Autodesk Fusion 360 part; units mm, degrees
note: some values were not read from the file. Chosen so that the rebuilt part matches the saved one: which bodies a step acts on.
(part 3 of 4)
ref_plane "WorkPlane163" through (39, 1188.0192, -25.0252) normal (1, 0, 0) x (0, 0, 1)
sketch "Sketch165" plane through (39, 1188.0192, -25.0252) normal (1, 0, 0) x (0, 0, 1)
  line L0 (0, 0) -> (-39.739, -22.9433) construction
  line L1 (-6.9433, 12.0262) -> (0, 0) construction
  line L2 (0, 0) -> (-2.9461, 0.7894) construction
  circle A0 centre (-2.9461, 0.7894) radius 3.05
  dimension "d1381" = 3.05
  constraint coincident L0.start L1.end
  constraint coincident L0.start A0
  measures "d1381" distance of L0.start L2.end
sweep "Sweep12''''" cut profiles "Sketch165" along 1 edges at (-419, -146.8099, -95.2685) section 1 sketch seen with x (1, 0, 0) y (0, 0, -1) z (0, 1, 0) at (-467, -121.7847, 1092.7507) on bodies 33 bodies 33 in component "Component''''''"
ref_plane "WorkPlane164" through (57, 1168.4645, 64.8206) normal (-1, 0, 0) x (0, 0, 1)
sketch "Sketch166" plane through (57, 1168.4645, 64.8206) normal (-1, 0, 0) x (0, 0, 1)
  line L0 (43.4745, -25.1) -> (0, 0) construction
  line L1 (0, 0) -> (9.1, 15.7617) construction
  line L2 (0, 0) -> (2.9461, 0.7894) construction
  circle A0 centre (2.9461, 0.7894) radius 3.05
  dimension "d1389" = 3.05
  constraint coincident L0.end L1.start
  constraint coincident L0.end A0
  measures "d1389" distance of L0.end L2.end
sweep "Sweep1''''" cut profiles "Sketch166" along 1 edges at (-27, -146.8099, -95.2685) section 1 sketch seen with x (1, 0, 0) y (0, 0, 1) z (0, -1, 0) at (-75, -81.9893, -1263.733) on bodies 31 bodies 31 in component "Component''''"
ref_plane "WorkPlane165" through (57, 1184.2262, 73.9206) normal (-1, 0, 0) x (0, 0, 1)
sketch "Sketch167" plane through (57, 1184.2262, 73.9206) normal (-1, 0, 0) x (0, 0, 1)
  line L0 (0, 0) -> (-6.9433, -12.0262) construction
  line L1 (43.4745, -25.1) -> (0, 0) construction
  line L2 (0, 0) -> (0.7894, -2.9461) construction
  circle A0 centre (0.7894, -2.9461) radius 3.05
  dimension "d1397" = 3.05
  constraint coincident L0.start L1.end
  constraint coincident L0.start A0
  measures "d1397" distance of L0.start L2.end
sweep "Sweep2''''" cut profiles "Sketch167" along 1 edges at (-27, -155.9099, -79.5068) section 1 sketch seen with x (1, 0, 0) y (0, 0, 1) z (0, -1, 0) at (-75, -81.9893, -1263.733) on bodies 31 bodies 31 in component "Component''''"
ref_plane "WorkPlane166" through (57, 1143.3645, 108.2951) normal (-1, 0, 0) x (0, 0, 1)
sketch "Sketch168" plane through (57, 1143.3645, 108.2951) normal (-1, 0, 0) x (0, 0, 1)
  line L0 (0, 0) -> (-39.739, 22.9433) construction
  line L1 (9.1, 15.7617) -> (0, 0) construction
  line L2 (0, 0) -> (-0.7894, 2.9461) construction
  circle A0 centre (-0.7894, 2.9461) radius 3.05
  dimension "d1405" = 3.05
  constraint coincident L0.start L1.end
  constraint coincident L0.start A0
  measures "d1405" distance of L0.start L2.end
sweep "Sweep3''''" cut profiles "Sketch168" along 1 edges at (-27, -190.2844, -120.3685) section 1 sketch seen with x (1, 0, 0) y (0, 0, 1) z (0, -1, 0) at (-75, -81.9893, -1263.733) on bodies 31 bodies 31 in component "Component''''"
ref_plane "WorkPlane167" through (57, 1159.1262, 117.3951) normal (-1, 0, 0) x (0, 0, 1)
sketch "Sketch169" plane through (57, 1159.1262, 117.3951) normal (-1, 0, 0) x (0, 0, 1)
  line L0 (0, 0) -> (-6.9433, -12.0262) construction
  line L1 (-39.739, 22.9433) -> (0, 0) construction
  line L2 (0, 0) -> (-2.9461, -0.7894) construction
  circle A0 centre (-2.9461, -0.7894) radius 3.05
  dimension "d1413" = 3.05
  constraint coincident L0.start L1.end
  constraint coincident L0.start A0
  measures "d1413" distance of L0.start L2.end
sweep "Sweep4''''" cut profiles "Sketch169" along 1 edges at (-27, -199.3844, -104.6068) section 1 sketch seen with x (1, 0, 0) y (0, 0, 1) z (0, -1, 0) at (-75, -81.9893, -1263.733) on bodies 31 bodies 31 in component "Component''''"
ref_plane "WorkPlane168" through (57, 1042.5615, 137.5107) normal (-1, 0, 0) x (0, 0, 1)
sketch "Sketch170" plane through (57, 1042.5615, 137.5107) normal (-1, 0, 0) x (0, 0, 1)
  line L0 (18.2, 0) -> (0, 0) construction
  line L1 (0, 0) -> (0, 50.2) construction
  line L2 (0, 0) -> (2.1567, 2.1567) construction
  circle A0 centre (2.1567, 2.1567) radius 3.05
  dimension "d1421" = 3.05
  constraint coincident L0.end L1.start
  constraint coincident L0.end A0
  measures "d1421" distance of L0.end L2.end
sweep "Sweep5'''''''''''''''''" cut profiles "Sketch170" along 1 edges at (-27, -219.5, -221.1715) section 1 sketch seen with x (1, 0, 0) y (0, 0, 1) z (0, -1, 0) at (-75, -81.9893, -1263.733) on bodies 31 bodies 31 in component "Component''''"
ref_plane "WorkPlane169" through (57, 1092.7615, 137.5107) normal (-1, 0, 0) x (0, 0, 1)
sketch "Sketch171" plane through (57, 1092.7615, 137.5107) normal (-1, 0, 0) x (0, 0, 1)
  line L0 (0, 0) -> (18.2, 0) construction
  line L1 (0, -45.8866) -> (0, 0) construction
  line L2 (0, 0) -> (2.1567, -2.1567) construction
  circle A0 centre (2.1567, -2.1567) radius 3.05
  dimension "d1429" = 3.05
  constraint coincident L0.start L1.end
  constraint coincident L0.start A0
  measures "d1429" distance of L0.start L2.end
sweep "Sweep6'''''''''''''''''" cut profiles "Sketch171" along 1 edges at (-27, -219.5, -170.9715) section 1 sketch seen with x (1, 0, 0) y (0, 0, 1) z (0, -1, 0) at (-75, -81.9893, -1263.733) on bodies 31 bodies 31 in component "Component''''"
ref_plane "WorkPlane170" through (57, 1092.7615, 155.7107) normal (-1, 0, 0) x (0, 0, 1)
sketch "Sketch172" plane through (57, 1092.7615, 155.7107) normal (-1, 0, 0) x (0, 0, 1)
  line L0 (0, 0) -> (0, -50.2) construction
  line L1 (-13.8866, 0) -> (0, 0) construction
  line L2 (0, 0) -> (-2.1567, -2.1567) construction
  circle A0 centre (-2.1567, -2.1567) radius 3.05
  dimension "d1437" = 3.05
  constraint coincident L0.start L1.end
  constraint coincident L0.start A0
  measures "d1437" distance of L0.start L2.end
sweep "Sweep7'''''''''''''''''" cut profiles "Sketch172" along 1 edges at (-27, -237.7, -170.9715) section 1 sketch seen with x (1, 0, 0) y (0, 0, 1) z (0, -1, 0) at (-75, -81.9893, -1263.733) on bodies 31 bodies 31 in component "Component''''"
ref_plane "WorkPlane171" through (57, 1042.5615, 155.7107) normal (-1, 0, 0) x (0, 0, 1)
sketch "Sketch173" plane through (57, 1042.5615, 155.7107) normal (-1, 0, 0) x (0, 0, 1)
  line L0 (0, 0) -> (0, 45.8866) construction
  line L1 (-13.8866, 0) -> (0, 0) construction
  line L2 (0, 0) -> (-2.1567, 2.1567) construction
  circle A0 centre (-2.1567, 2.1567) radius 3.05
  dimension "d1445" = 3.05
  constraint coincident L0.start L1.end
  constraint coincident L0.start A0
  measures "d1445" distance of L0.start L2.end
sweep "Sweep8'''''''''''''''''" cut profiles "Sketch173" along 1 edges at (-27, -237.7, -221.1715) section 1 sketch seen with x (1, 0, 0) y (0, 0, 1) z (0, -1, 0) at (-75, -81.9893, -1263.733) on bodies 31 bodies 31 in component "Component''''"
ref_plane "WorkPlane172" through (57, 1159.1262, 175.8264) normal (-1, 0, 0) x (0, 0, 1)
sketch "Sketch174" plane through (57, 1159.1262, 175.8264) normal (-1, 0, 0) x (0, 0, 1)
  line L0 (9.1, -15.7617) -> (0, 0) construction
  line L1 (0, 0) -> (43.4745, 25.1) construction
  line L2 (0, 0) -> (2.9461, -0.7894) construction
  circle A0 centre (2.9461, -0.7894) radius 3.05
  dimension "d1453" = 3.05
  constraint coincident L0.end L1.start
  constraint coincident L0.end A0
  measures "d1453" distance of L0.end L2.end
sweep "Sweep9'''''" cut profiles "Sketch174" along 1 edges at (-27, -257.8156, -104.6068) section 1 sketch seen with x (1, 0, 0) y (0, 0, 1) z (0, -1, 0) at (-75, -81.9893, -1263.733) on bodies 31 bodies 31 in component "Component''''"
ref_plane "WorkPlane173" through (57, 1143.3645, 184.9264) normal (-1, 0, 0) x (0, 0, 1)
sketch "Sketch175" plane through (57, 1143.3645, 184.9264) normal (-1, 0, 0) x (0, 0, 1)
  line L0 (43.4745, 25.1) -> (0, 0) construction
  line L1 (0, 0) -> (-6.9433, 12.0262) construction
  line L2 (0, 0) -> (0.7894, 2.9461) construction
  circle A0 centre (0.7894, 2.9461) radius 3.05
  dimension "d1461" = 3.05
  constraint coincident L0.end L1.start
  constraint coincident L0.end A0
  measures "d1461" distance of L0.end L2.end
sweep "Sweep10'''''" cut profiles "Sketch175" along 1 edges at (-27, -266.9156, -120.3685) section 1 sketch seen with x (1, 0, 0) y (0, 0, 1) z (0, -1, 0) at (-75, -81.9893, -1263.733) on bodies 31 bodies 31 in component "Component''''"
ref_plane "WorkPlane174" through (57, 1184.2262, 219.3009) normal (-1, 0, 0) x (0, 0, 1)
sketch "Sketch176" plane through (57, 1184.2262, 219.3009) normal (-1, 0, 0) x (0, 0, 1)
  line L0 (0, 0) -> (9.1, -15.7617) construction
  line L1 (-39.739, -22.9433) -> (0, 0) construction
  line L2 (0, 0) -> (-0.7894, -2.9461) construction
  circle A0 centre (-0.7894, -2.9461) radius 3.05
  dimension "d1469" = 3.05
  constraint coincident L0.start L1.end
  constraint coincident L0.start A0
  measures "d1469" distance of L0.start L2.end
sweep "Sweep11'''''" cut profiles "Sketch176" along 1 edges at (-27, -301.2901, -79.5068) section 1 sketch seen with x (1, 0, 0) y (0, 0, 1) z (0, -1, 0) at (-75, -81.9893, -1263.733) on bodies 31 bodies 31 in component "Component''''"
ref_plane "WorkPlane175" through (57, 1168.4645, 228.4009) normal (-1, 0, 0) x (0, 0, 1)
sketch "Sketch177" plane through (57, 1168.4645, 228.4009) normal (-1, 0, 0) x (0, 0, 1)
  line L0 (0, 0) -> (-39.739, -22.9433) construction
  line L1 (-6.9433, 12.0262) -> (0, 0) construction
  line L2 (0, 0) -> (-2.9461, 0.7894) construction
  circle A0 centre (-2.9461, 0.7894) radius 3.05
  dimension "d1477" = 3.05
  constraint coincident L0.start L1.end
  constraint coincident L0.start A0
  measures "d1477" distance of L0.start L2.end
sweep "Sweep12'''''" cut profiles "Sketch177" along 1 edges at (-27, -310.3901, -95.2685) section 1 sketch seen with x (1, 0, 0) y (0, 0, 1) z (0, -1, 0) at (-75, -81.9893, -1263.733) on bodies 31 bodies 31 in component "Component''''"
ref_plane "WorkPlane176" through (57, 1188.0193, 318.2466) normal (-1, 0, 0) x (0, 0.866025, 0.5)
sketch "Sketch178" plane through (57, 1188.0193, 318.2466) normal (-1, 0, 0) x (0, 0.866025, 0.5)
  line L0 (-9.1, -15.7617) -> (0, 0) construction
  line L1 (0, 0) -> (43.4745, -25.1) construction
  line L2 (0, 0) -> (0.7894, -2.9461) construction
  circle A0 centre (0.7894, -2.9461) radius 3.05
  dimension "d1485" = 3.05
  constraint coincident L0.end L1.start
  constraint coincident L0.end A0
  measures "d1485" distance of L0.end L2.end
sweep "Sweep1'''''" cut profiles "Sketch178" along 1 edges at (-27, 73.1741, 316.2364) section 1 sketch seen with x (1, 0, 0) y (0, -0.866025, 0.5) z (0, -0.5, -0.866025) at (-75, 1261.1523, -2.1636) on bodies 37 bodies 37 in component "Component''''''''''"
ref_plane "WorkPlane177" through (57, 1172.2576, 327.3466) normal (-1, 0, 0) x (0, 0.866025, 0.5)
sketch "Sketch179" plane through (57, 1172.2576, 327.3466) normal (-1, 0, 0) x (0, 0.866025, 0.5)
  line L0 (0, 0) -> (6.9433, 12.0262) construction
  line L1 (43.4745, -25.1) -> (0, 0) construction
  line L2 (0, 0) -> (2.9461, 0.7894) construction
  circle A0 centre (2.9461, 0.7894) radius 3.05
  dimension "d1493" = 3.05
  constraint coincident L0.start L1.end
  constraint coincident L0.start A0
  measures "d1493" distance of L0.start L2.end
sweep "Sweep2'''''" cut profiles "Sketch179" along 1 edges at (-27, 82.2741, 300.4748) section 1 sketch seen with x (1, 0, 0) y (0, -0.866025, 0.5) z (0, -0.5, -0.866025) at (-75, 1261.1523, -2.1636) on bodies 37 bodies 37 in component "Component''''''''''"
ref_plane "WorkPlane178" through (57, 1213.1193, 361.721) normal (-1, 0, 0) x (0, 0.866025, 0.5)
sketch "Sketch180" plane through (57, 1213.1193, 361.721) normal (-1, 0, 0) x (0, 0.866025, 0.5)
  line L0 (0, 0) -> (-9.1, -15.7617) construction
  line L1 (-39.739, 22.9433) -> (0, 0) construction
  line L2 (0, 0) -> (-2.9461, -0.7894) construction
  circle A0 centre (-2.9461, -0.7894) radius 3.05
  dimension "d1501" = 3.05
  constraint coincident L0.start L1.end
  constraint coincident L0.start A0
  measures "d1501" distance of L0.start L2.end
sweep "Sweep3'''''" cut profiles "Sketch180" along 1 edges at (-27, 29.6997, 291.1364) section 1 sketch seen with x (1, 0, 0) y (0, -0.866025, 0.5) z (0, -0.5, -0.866025) at (-75, 1261.1523, -2.1636) on bodies 37 bodies 37 in component "Component''''''''''"
ref_plane "WorkPlane179" through (57, 1197.3576, 370.821) normal (-1, 0, 0) x (0, 0.866025, 0.5)
sketch "Sketch181" plane through (57, 1197.3576, 370.821) normal (-1, 0, 0) x (0, 0.866025, 0.5)
  line L0 (0, 0) -> (-39.739, 22.9433) construction
  line L1 (6.9433, 12.0262) -> (0, 0) construction
  line L2 (0, 0) -> (-0.7894, 2.9461) construction
  circle A0 centre (-0.7894, 2.9461) radius 3.05
  dimension "d1509" = 3.05
  constraint coincident L0.start L1.end
  constraint coincident L0.start A0
  measures "d1509" distance of L0.start L2.end
sweep "Sweep4'''''" cut profiles "Sketch181" along 1 edges at (-27, 38.7997, 275.3748) section 1 sketch seen with x (1, 0, 0) y (0, -0.866025, 0.5) z (0, -0.5, -0.866025) at (-75, 1261.1523, -2.1636) on bodies 37 bodies 37 in component "Component''''''''''"
ref_plane "WorkPlane180" through (57, 1313.9223, 390.9367) normal (-1, 0, 0) x (0, 0.866025, 0.5)
sketch "Sketch182" plane through (57, 1313.9223, 390.9367) normal (-1, 0, 0) x (0, 0.866025, 0.5)
  line L0 (0, 0) -> (9.1, -15.7617) construction
  line L1 (-43.4745, -25.1) -> (0, 0) construction
  line L2 (0, 0) -> (-0.7894, -2.9461) construction
  circle A0 centre (-0.7894, -2.9461) radius 3.05
  dimension "d1517" = 3.05
  constraint coincident L0.start L1.end
  constraint coincident L0.start A0
  measures "d1517" distance of L0.start L2.end
sweep "Sweep5''''''''''''''''''" cut profiles "Sketch182" along 1 edges at (-27, -72.2061, 316.2364) section 1 sketch seen with x (1, 0, 0) y (0, -0.866025, 0.5) z (0, -0.5, -0.866025) at (-75, 1261.1523, -2.1636) on bodies 37 bodies 37 in component "Component''''''''''"
ref_plane "WorkPlane181" through (57, 1263.7223, 390.9367) normal (-1, 0, 0) x (0, 0.866025, 0.5)
sketch "Sketch183" plane through (57, 1263.7223, 390.9367) normal (-1, 0, 0) x (0, 0.866025, 0.5)
  line L0 (0, 0) -> (39.739, 22.9433) construction
  line L1 (9.1, -15.7617) -> (0, 0) construction
  line L2 (0, 0) -> (2.9461, -0.7894) construction
  circle A0 centre (2.9461, -0.7894) radius 3.05
  dimension "d1525" = 3.05
  constraint coincident L0.start L1.end
  constraint coincident L0.start A0
  measures "d1525" distance of L0.start L2.end
sweep "Sweep6''''''''''''''''''" cut profiles "Sketch183" along 1 edges at (-27, -28.7316, 291.1364) section 1 sketch seen with x (1, 0, 0) y (0, -0.866025, 0.5) z (0, -0.5, -0.866025) at (-75, 1261.1523, -2.1636) on bodies 37 bodies 37 in component "Component''''''''''"
ref_plane "WorkPlane182" through (57, 1313.9223, 409.1367) normal (-1, 0, 0) x (0, 0.866025, 0.5)
sketch "Sketch184" plane through (57, 1313.9223, 409.1367) normal (-1, 0, 0) x (0, 0.866025, 0.5)
  line L0 (0, 0) -> (-6.9433, 12.0262) construction
  line L1 (-43.4745, -25.1) -> (0, 0) construction
  line L2 (0, 0) -> (-2.9461, 0.7894) construction
  circle A0 centre (-2.9461, 0.7894) radius 3.05
  dimension "d1533" = 3.05
  constraint coincident L0.start L1.end
  constraint coincident L0.start A0
  measures "d1533" distance of L0.start L2.end
sweep "Sweep7''''''''''''''''''" cut profiles "Sketch184" along 1 edges at (-27, -81.3061, 300.4748) section 1 sketch seen with x (1, 0, 0) y (0, -0.866025, 0.5) z (0, -0.5, -0.866025) at (-75, 1261.1523, -2.1636) on bodies 37 bodies 37 in component "Component''''''''''"
ref_plane "WorkPlane183" through (57, 1263.7223, 409.1367) normal (-1, 0, 0) x (0, 0.866025, 0.5)
sketch "Sketch185" plane through (57, 1263.7223, 409.1367) normal (-1, 0, 0) x (0, 0.866025, 0.5)
  line L0 (0, 0) -> (-6.9433, 12.0262) construction
  line L1 (39.739, 22.9433) -> (0, 0) construction
  line L2 (0, 0) -> (0.7894, 2.9461) construction
  circle A0 centre (0.7894, 2.9461) radius 3.05
  dimension "d1541" = 3.05
  constraint coincident L0.start L1.end
  constraint coincident L0.start A0
  measures "d1541" distance of L0.start L2.end
sweep "Sweep8''''''''''''''''''" cut profiles "Sketch185" along 1 edges at (-27, -37.8316, 275.3748) section 1 sketch seen with x (1, 0, 0) y (0, -0.866025, 0.5) z (0, -0.5, -0.866025) at (-75, 1261.1523, -2.1636) on bodies 37 bodies 37 in component "Component''''''''''"
ref_plane "WorkPlane184" through (57, 1197.3576, 429.2523) normal (-1, 0, 0) x (0, 0.866025, 0.5)
sketch "Sketch186" plane through (57, 1197.3576, 429.2523) normal (-1, 0, 0) x (0, 0.866025, 0.5)
  line L0 (0, 0) -> (18.2, 0) construction
  line L1 (0, -50.2) -> (0, 0) construction
  line L2 (0, 0) -> (2.1567, -2.1567) construction
  circle A0 centre (2.1567, -2.1567) radius 3.05
  dimension "d1549" = 3.05
  constraint coincident L0.start L1.end
  constraint coincident L0.start A0
  measures "d1549" distance of L0.start L2.end
sweep "Sweep9''''''" cut profiles "Sketch186" along 1 edges at (-27, 9.584, 224.7718) section 1 sketch seen with x (1, 0, 0) y (0, -0.866025, 0.5) z (0, -0.5, -0.866025) at (-75, 1261.1523, -2.1636) on bodies 37 bodies 37 in component "Component''''''''''"
ref_plane "WorkPlane185" through (57, 1213.1193, 438.3523) normal (-1, 0, 0) x (0, 0.866025, 0.5)
sketch "Sketch187" plane through (57, 1213.1193, 438.3523) normal (-1, 0, 0) x (0, 0.866025, 0.5)
  line L0 (0, 0) -> (0, -50.2) construction
  line L1 (-13.8866, 0) -> (0, 0) construction
  line L2 (0, 0) -> (-2.1567, -2.1567) construction
  circle A0 centre (-2.1567, -2.1567) radius 3.05
  dimension "d1557" = 3.05
  constraint coincident L0.start L1.end
  constraint coincident L0.start A0
  measures "d1557" distance of L0.start L2.end
sweep "Sweep10''''''" cut profiles "Sketch187" along 1 edges at (-27, -8.616, 224.7718) section 1 sketch seen with x (1, 0, 0) y (0, -0.866025, 0.5) z (0, -0.5, -0.866025) at (-75, 1261.1523, -2.1636) on bodies 37 bodies 37 in component "Component''''''''''"
ref_plane "WorkPlane186" through (57, 1172.2576, 472.7268) normal (-1, 0, 0) x (0, 0.866025, 0.5)
sketch "Sketch188" plane through (57, 1172.2576, 472.7268) normal (-1, 0, 0) x (0, 0.866025, 0.5)
  line L0 (18.2, 0) -> (0, 0) construction
  line L1 (0, 0) -> (0, 45.8866) construction
  line L2 (0, 0) -> (2.1567, 2.1567) construction
  circle A0 centre (2.1567, 2.1567) radius 3.05
  dimension "d1565" = 3.05
  constraint coincident L0.end L1.start
  constraint coincident L0.end A0
  measures "d1565" distance of L0.end L2.end
sweep "Sweep11''''''" cut profiles "Sketch188" along 1 edges at (-27, 9.584, 174.5718) section 1 sketch seen with x (1, 0, 0) y (0, -0.866025, 0.5) z (0, -0.5, -0.866025) at (-75, 1261.1523, -2.1636) on bodies 37 bodies 37 in component "Component''''''''''"
ref_plane "WorkPlane187" through (57, 1188.0193, 481.8268) normal (-1, 0, 0) x (0, 0.866025, 0.5)
sketch "Sketch189" plane through (57, 1188.0193, 481.8268) normal (-1, 0, 0) x (0, 0.866025, 0.5)
  line L0 (0, 0) -> (-13.8866, 0) construction
  line L1 (0, 45.8866) -> (0, 0) construction
  line L2 (0, 0) -> (-2.1567, 2.1567) construction
  circle A0 centre (-2.1567, 2.1567) radius 3.05
  dimension "d1573" = 3.05
  constraint coincident L0.start L1.end
  constraint coincident L0.start A0
  measures "d1573" distance of L0.start L2.end
sweep "Sweep12''''''" cut profiles "Sketch189" along 1 edges at (-27, -8.616, 174.5718) section 1 sketch seen with x (1, 0, 0) y (0, -0.866025, 0.5) z (0, -0.5, -0.866025) at (-75, 1261.1523, -2.1636) on bodies 37 bodies 37 in component "Component''''''''''"
ref_plane "WorkPlane188" through (39, 1168.4646, 571.6732) normal (1, 0, 0) x (0, 0.866025, 0.5)
sketch "Sketch190" plane through (39, 1168.4646, 571.6732) normal (1, 0, 0) x (0, 0.866025, 0.5)
  line L0 (18.2, 0) -> (0, 0) construction
  line L1 (0, 0) -> (0, 50.2) construction
  line L2 (0, 0) -> (2.1567, 2.1567) construction
  circle A0 centre (2.1567, 2.1567) radius 3.05
  dimension "d1581" = 3.05
  constraint coincident L0.end L1.start
  constraint coincident L0.end A0
  measures "d1581" distance of L0.end L2.end
sweep "Sweep1''''''" cut profiles "Sketch190" along 1 edges at (-419, -8.616, 174.5718) section 1 sketch seen with x (1, 0, 0) y (0, 0.866025, -0.5) z (0, 0.5, 0.866025) at (-467, -1306.3726, 263.7206) on bodies 39 bodies 39 in component "Component''''''''''''"
ref_plane "WorkPlane189" through (39, 1184.2262, 580.7732) normal (1, 0, 0) x (0, 0.866025, 0.5)
sketch "Sketch191" plane through (39, 1184.2262, 580.7732) normal (1, 0, 0) x (0, 0.866025, 0.5)
  line L0 (0, 50.2) -> (0, 0) construction
  line L1 (0, 0) -> (-13.8866, 0) construction
  line L2 (0, 0) -> (-2.1567, 2.1567) construction
  circle A0 centre (-2.1567, 2.1567) radius 3.05
  dimension "d1589" = 3.05
  constraint coincident L0.end L1.start
  constraint coincident L0.end A0
  measures "d1589" distance of L0.end L2.end
sweep "Sweep2''''''" cut profiles "Sketch191" along 1 edges at (-419, 9.584, 174.5718) section 1 sketch seen with x (1, 0, 0) y (0, 0.866025, -0.5) z (0, 0.5, 0.866025) at (-467, -1306.3726, 263.7206) on bodies 39 bodies 39 in component "Component''''''''''''"
ref_plane "WorkPlane190" through (39, 1143.3646, 615.1477) normal (1, 0, 0) x (0, 0.866025, 0.5)
sketch "Sketch192" plane through (39, 1143.3646, 615.1477) normal (1, 0, 0) x (0, 0.866025, 0.5)
  line L0 (0, 0) -> (18.2, 0) construction
  line L1 (0, -45.8866) -> (0, 0) construction
  line L2 (0, 0) -> (2.1567, -2.1567) construction
  circle A0 centre (2.1567, -2.1567) radius 3.05
  dimension "d1597" = 3.05
  constraint coincident L0.start L1.end
  constraint coincident L0.start A0
  measures "d1597" distance of L0.start L2.end
sweep "Sweep3''''''" cut profiles "Sketch192" along 1 edges at (-419, -8.616, 224.7718) section 1 sketch seen with x (1, 0, 0) y (0, 0.866025, -0.5) z (0, 0.5, 0.866025) at (-467, -1306.3726, 263.7206) on bodies 39 bodies 39 in component "Component''''''''''''"
ref_plane "WorkPlane191" through (39, 1159.1262, 624.2477) normal (1, 0, 0) x (0, 0.866025, 0.5)
sketch "Sketch193" plane through (39, 1159.1262, 624.2477) normal (1, 0, 0) x (0, 0.866025, 0.5)
  line L0 (0, 0) -> (-13.8866, 0) construction
  line L1 (0, -45.8866) -> (0, 0) construction
  line L2 (0, 0) -> (-2.1567, -2.1567) construction
  circle A0 centre (-2.1567, -2.1567) radius 3.05
  dimension "d1605" = 3.05
  constraint coincident L0.start L1.end
  constraint coincident L0.start A0
  measures "d1605" distance of L0.start L2.end
sweep "Sweep4''''''" cut profiles "Sketch193" along 1 edges at (-419, 9.584, 224.7718) section 1 sketch seen with x (1, 0, 0) y (0, 0.866025, -0.5) z (0, 0.5, 0.866025) at (-467, -1306.3726, 263.7206) on bodies 39 bodies 39 in component "Component''''''''''''"
ref_plane "WorkPlane192" through (39, 1092.7616, 644.3633) normal (1, 0, 0) x (0, 0.866025, 0.5)
sketch "Sketch194" plane through (39, 1092.7616, 644.3633) normal (1, 0, 0) x (0, 0.866025, 0.5)
  line L0 (9.1, 15.7617) -> (0, 0) construction
  line L1 (0, 0) -> (-43.4745, 25.1) construction
  line L2 (0, 0) -> (-0.7894, 2.9461) construction
  circle A0 centre (-0.7894, 2.9461) radius 3.05
  dimension "d1613" = 3.05
  constraint coincident L0.end L1.start
  constraint coincident L0.end A0
  measures "d1613" distance of L0.end L2.end
sweep "Sweep5'''''''''''''''''''" cut profiles "Sketch194" along 1 edges at (-419, -37.8316, 275.3748) section 1 sketch seen with x (1, 0, 0) y (0, 0.866025, -0.5) z (0, 0.5, 0.866025) at (-467, -1306.3726, 263.7206) on bodies 39 bodies 39 in component "Component''''''''''''"
ref_plane "WorkPlane193" through (39, 1042.5616, 644.3633) normal (1, 0, 0) x (0, 0.866025, 0.5)
sketch "Sketch195" plane through (39, 1042.5616, 644.3633) normal (1, 0, 0) x (0, 0.866025, 0.5)
  line L0 (0, 0) -> (39.739, -22.9433) construction
  line L1 (9.1, 15.7617) -> (0, 0) construction
  line L2 (0, 0) -> (2.9461, 0.7894) construction
  circle A0 centre (2.9461, 0.7894) radius 3.05
  dimension "d1621" = 3.05
  constraint coincident L0.start L1.end
  constraint coincident L0.start A0
  measures "d1621" distance of L0.start L2.end
sweep "Sweep6'''''''''''''''''''" cut profiles "Sketch195" along 1 edges at (-419, -81.3061, 300.4748) section 1 sketch seen with x (1, 0, 0) y (0, 0.866025, -0.5) z (0, 0.5, 0.866025) at (-467, -1306.3726, 263.7206) on bodies 39 bodies 39 in component "Component''''''''''''"
ref_plane "WorkPlane194" through (39, 1042.5616, 662.5633) normal (1, 0, 0) x (0, 0.866025, 0.5)
sketch "Sketch196" plane through (39, 1042.5616, 662.5633) normal (1, 0, 0) x (0, 0.866025, 0.5)
  line L0 (0, 0) -> (-6.9433, -12.0262) construction
  line L1 (43.4745, -25.1) -> (0, 0) construction
  line L2 (0, 0) -> (0.7894, -2.9461) construction
  circle A0 centre (0.7894, -2.9461) radius 3.05
  dimension "d1629" = 3.05
  constraint coincident L0.start L1.end
  constraint coincident L0.start A0
  measures "d1629" distance of L0.start L2.end
sweep "Sweep7'''''''''''''''''''" cut profiles "Sketch196" along 1 edges at (-419, -72.2061, 316.2364) section 1 sketch seen with x (1, 0, 0) y (0, 0.866025, -0.5) z (0, 0.5, 0.866025) at (-467, -1306.3726, 263.7206) on bodies 39 bodies 39 in component "Component''''''''''''"
ref_plane "WorkPlane195" through (39, 1092.7616, 662.5633) normal (1, 0, 0) x (0, 0.866025, 0.5)
sketch "Sketch197" plane through (39, 1092.7616, 662.5633) normal (1, 0, 0) x (0, 0.866025, 0.5)
  line L0 (0, 0) -> (-6.9433, -12.0262) construction
  line L1 (-39.739, 22.9433) -> (0, 0) construction
  line L2 (0, 0) -> (-2.9461, -0.7894) construction
  circle A0 centre (-2.9461, -0.7894) radius 3.05
  dimension "d1637" = 3.05
  constraint coincident L0.start L1.end
  constraint coincident L0.start A0
  measures "d1637" distance of L0.start L2.end
sweep "Sweep8'''''''''''''''''''" cut profiles "Sketch197" along 1 edges at (-419, -28.7316, 291.1364) section 1 sketch seen with x (1, 0, 0) y (0, 0.866025, -0.5) z (0, 0.5, 0.866025) at (-467, -1306.3726, 263.7206) on bodies 39 bodies 39 in component "Component''''''''''''"
ref_plane "WorkPlane196" through (39, 1159.1262, 682.679) normal (1, 0, 0) x (0, 0.866025, 0.5)
sketch "Sketch198" plane through (39, 1159.1262, 682.679) normal (1, 0, 0) x (0, 0.866025, 0.5)
  line L0 (0, 0) -> (-9.1, 15.7617) construction
  line L1 (43.4745, 25.1) -> (0, 0) construction
  line L2 (0, 0) -> (0.7894, 2.9461) construction
  circle A0 centre (0.7894, 2.9461) radius 3.05
  dimension "d1645" = 3.05
  constraint coincident L0.start L1.end
  constraint coincident L0.start A0
  measures "d1645" distance of L0.start L2.end
sweep "Sweep9'''''''" cut profiles "Sketch198" along 1 edges at (-419, 38.7997, 275.3748) section 1 sketch seen with x (1, 0, 0) y (0, 0.866025, -0.5) z (0, 0.5, 0.866025) at (-467, -1306.3726, 263.7206) on bodies 39 bodies 39 in component "Component''''''''''''"
ref_plane "WorkPlane197" through (39, 1143.3646, 691.779) normal (1, 0, 0) x (0, 0.866025, 0.5)
sketch "Sketch199" plane through (39, 1143.3646, 691.779) normal (1, 0, 0) x (0, 0.866025, 0.5)
  line L0 (0, 0) -> (6.9433, -12.0262) construction
  line L1 (43.4745, 25.1) -> (0, 0) construction
  line L2 (0, 0) -> (2.9461, -0.7894) construction
  circle A0 centre (2.9461, -0.7894) radius 3.05
  dimension "d1653" = 3.05
  constraint coincident L0.start L1.end
  constraint coincident L0.start A0
  measures "d1653" distance of L0.start L2.end
sweep "Sweep10'''''''" cut profiles "Sketch199" along 1 edges at (-419, 29.6997, 291.1364) section 1 sketch seen with x (1, 0, 0) y (0, 0.866025, -0.5) z (0, 0.5, 0.866025) at (-467, -1306.3726, 263.7206) on bodies 39 bodies 39 in component "Component''''''''''''"
ref_plane "WorkPlane198" through (39, 1184.2262, 726.1534) normal (1, 0, 0) x (0, 0.866025, 0.5)
sketch "Sketch200" plane through (39, 1184.2262, 726.1534) normal (1, 0, 0) x (0, 0.866025, 0.5)
  line L0 (-9.1, 15.7617) -> (0, 0) construction
  line L1 (0, 0) -> (-39.739, -22.9433) construction
  line L2 (0, 0) -> (-2.9461, 0.7894) construction
  circle A0 centre (-2.9461, 0.7894) radius 3.05
  dimension "d1661" = 3.05
  constraint coincident L0.end L1.start
  constraint coincident L0.end A0
  measures "d1661" distance of L0.end L2.end
sweep "Sweep11'''''''" cut profiles "Sketch200" along 1 edges at (-419, 82.2741, 300.4748) section 1 sketch seen with x (1, 0, 0) y (0, 0.866025, -0.5) z (0, 0.5, 0.866025) at (-467, -1306.3726, 263.7206) on bodies 39 bodies 39 in component "Component''''''''''''"
ref_plane "WorkPlane199" through (39, 1168.4646, 735.2534) normal (1, 0, 0) x (0, 0.866025, 0.5)
sketch "Sketch201" plane through (39, 1168.4646, 735.2534) normal (1, 0, 0) x (0, 0.866025, 0.5)
  line L0 (0, 0) -> (-39.739, -22.9433) construction
  line L1 (6.9433, -12.0262) -> (0, 0) construction
  line L2 (0, 0) -> (-0.7894, -2.9461) construction
  circle A0 centre (-0.7894, -2.9461) radius 3.05
  dimension "d1669" = 3.05
  constraint coincident L0.start L1.end
  constraint coincident L0.start A0
  measures "d1669" distance of L0.start L2.end
sweep "Sweep12'''''''" cut profiles "Sketch201" along 1 edges at (-419, 73.1741, 316.2364) section 1 sketch seen with x (1, 0, 0) y (0, 0.866025, -0.5) z (0, 0.5, 0.866025) at (-467, -1306.3726, 263.7206) on bodies 39 bodies 39 in component "Component''''''''''''"
sketch "Sketch5" plane through (57, 0, 0) normal (1, 0, 0) x (0, 1, 0)
  arc A0 (1476.8936, -1070.6601) -> (1476.8936, -1018.6986) centre (1461.8936, -1044.6793) ccw
  line L0 (1476.8936, -1018.6986) -> (775, -613.4601)
  arc A1 (775, -613.4601) -> (730, -639.4408) centre (760, -639.4408) ccw
  line L1 (730, -639.4408) -> (730, -1449.9178)
  arc A2 (730, -1449.9178) -> (775, -1475.8986) centre (760, -1449.9178) ccw
  line L2 (775, -1475.8986) -> (1476.8936, -1070.6601)
  line L3 (1042.8501, -969.5804) -> (1034.5593, -964.7937)
  line L4 (1032.9805, -958.9016) -> (1073.7672, -888.257)
  line L5 (1079.6593, -886.6783) -> (1087.9501, -891.4649)
  line L6 (1089.5289, -897.357) -> (1048.7422, -968.0016)
  line L7 (904.4842, -1039.8927) -> (904.4842, -1049.466)
  line L8 (900.1708, -1053.7793) -> (818.5975, -1053.7793)
  line L9 (814.2842, -1049.466) -> (814.2842, -1039.8927)
  line L10 (818.5975, -1035.5793) -> (900.1708, -1035.5793)
  line L11 (1034.5593, -1124.5649) -> (1042.8501, -1119.7783)
  line L12 (1048.7422, -1121.357) -> (1089.5289, -1192.0016)
  line L13 (1087.9501, -1197.8937) -> (1079.6593, -1202.6804)
  line L14 (1073.7672, -1201.1016) -> (1032.9805, -1130.457)
  line L15 (1344.4624, -1368.5013) -> (1336.1717, -1363.7146)
  line L16 (1334.5929, -1357.8225) -> (1355.3796, -1321.8189)
  line L17 (1361.2717, -1320.2401) -> (1369.5624, -1325.0268)
  line L18 (1371.1412, -1330.9189) -> (1350.3546, -1366.9225)
  line L19 (1336.1717, -1214.021) -> (1344.4624, -1209.2344)
  line L20 (1350.3546, -1210.8132) -> (1371.1412, -1246.8167)
  line L21 (1369.5624, -1252.7088) -> (1361.2717, -1257.4955)
  line L22 (1355.3796, -1255.9167) -> (1334.5929, -1219.9132)
  line L23 (1474.1009, -1284.0812) -> (1474.1009, -1293.6545)
  line L24 (1469.7876, -1297.9678) -> (1428.2143, -1297.9678)
  line L25 (1423.9009, -1293.6545) -> (1423.9009, -1284.0812)
  line L26 (1428.2143, -1279.7678) -> (1469.7876, -1279.7678)
  arc A3 (1183.9472, -1262.8871) -> (1183.9472, -1314.8486) centre (1198.9472, -1288.8678) ccw
  line L27 (1183.9472, -1314.8486) -> (1462.894, -1475.8986)
  arc A4 (1462.894, -1475.8986) -> (1507.894, -1449.9178) centre (1477.894, -1449.9178) ccw
  line L28 (1507.894, -1449.9178) -> (1507.894, -1127.8178)
  arc A5 (1507.894, -1127.8178) -> (1462.894, -1101.837) centre (1477.894, -1127.8178) ccw
  line L29 (1462.894, -1101.837) -> (1183.9472, -1262.8871)
  line L30 (1527.8941, -1471.2) -> (1557.4738, -1471.2)
  line L31 (1645.6802, -1471.2) -> (1645.6802, -1097.2)
  line L32 (1645.6802, -1097.2) -> (1616.1005, -1097.2)
  line L33 (1611.7871, -1092.8866) -> (1611.7871, -1079.2)
  line L34 (1611.7871, -1079.2) -> (1561.7871, -1079.2)
  line L35 (1561.7871, -1079.2) -> (1561.7871, -1092.8866)
  line L36 (1557.4738, -1097.2) -> (1527.8941, -1097.2)
  line L37 (1527.8941, -1097.2) -> (1527.8941, -1471.2)
  line L38 (1561.7871, -1475.5133) -> (1561.7871, -1489.2)
  line L39 (1561.7871, -1489.2) -> (1611.7871, -1489.2)
  line L40 (1611.7871, -1489.2) -> (1611.7871, -1475.5133)
  line L41 (1557.4739, -667.2) -> (1527.8941, -667.2)
  line L42 (1527.8941, -667.2) -> (1527.8941, -1041.2)
  line L43 (1527.8941, -1041.2) -> (1557.4739, -1041.2)
  line L44 (1561.7872, -1045.5133) -> (1561.7872, -1059.2)
  line L45 (1561.7872, -1059.2) -> (1611.7872, -1059.2)
  line L46 (1611.7872, -1059.2) -> (1611.7872, -1045.5133)
  line L47 (1616.1006, -1041.2) -> (1645.6803, -1041.2)
  line L48 (1645.6803, -1041.2) -> (1645.6803, -667.2)
  line L49 (1611.7872, -662.8866) -> (1611.7872, -649.2)
  line L50 (1611.7872, -649.2) -> (1561.7872, -649.2)
  line L51 (1561.7872, -649.2) -> (1561.7872, -662.8866)
  line L52 (1390.1081, -937.046) -> (1419.6879, -937.046)
  line L53 (1507.8943, -937.046) -> (1507.8943, -563.046)
  line L54 (1507.8943, -563.046) -> (1478.3146, -563.046)
  line L55 (1474.0012, -558.7326) -> (1474.0012, -545.046)
  line L56 (1474.0012, -545.046) -> (1424.0012, -545.046)
  line L57 (1424.0012, -545.046) -> (1424.0012, -558.7326)
  line L58 (1419.6879, -563.046) -> (1390.1081, -563.046)
  line L59 (1390.1081, -563.046) -> (1390.1081, -937.046)
  line L60 (1424.0012, -941.3593) -> (1424.0012, -955.046)
  line L61 (1424.0012, -955.046) -> (1474.0012, -955.046)
  line L62 (1474.0012, -955.046) -> (1474.0012, -941.3593)
  line L63 (1217.2116, -740.7254) -> (1225.5023, -735.9387)
  line L64 (1231.3944, -737.5175) -> (1272.1811, -808.1621)
  line L65 (1270.6023, -814.0542) -> (1262.3116, -818.8409)
  line L66 (1256.4194, -817.2621) -> (1215.6328, -746.6175)
  line L67 (1001.2498, -651.7398) -> (1082.823, -651.7398)
  line L68 (1087.1364, -656.0531) -> (1087.1364, -665.6264)
  line L69 (1082.823, -669.9398) -> (1001.2498, -669.9398)
  line L70 (996.9364, -665.6264) -> (996.9364, -656.0531)
  line L71 (1225.5023, -585.7409) -> (1217.2116, -580.9542)
  line L72 (1215.6328, -575.0621) -> (1256.4194, -504.4175)
  line L73 (1262.3116, -502.8387) -> (1270.6023, -507.6254)
  line L74 (1272.1811, -513.5175) -> (1231.3944, -584.1621)
  line L75 (1300.8048, -893.9398) -> (1316.3932, -884.9398)
  line L76 (1316.3932, -884.9398) -> (1316.3932, -436.7398)
  line L77 (1316.3932, -436.7398) -> (1300.8048, -427.7398)
  line L78 (1300.8048, -427.7398) -> (912.6522, -651.8398)
  line L79 (912.6522, -651.8398) -> (912.6522, -669.8398)
  line L80 (912.6522, -669.8398) -> (1300.8048, -893.9398)
  line L81 (1535.0811, -169.0459) -> (1505.5014, -169.0459)
  line L82 (1505.5014, -169.0459) -> (1505.5014, -543.0459)
  line L83 (1505.5014, -543.0459) -> (1535.0811, -543.0459)
  line L84 (1539.3944, -547.3592) -> (1539.3944, -561.0459)
  line L85 (1539.3944, -561.0459) -> (1589.3944, -561.0459)
  line L86 (1589.3944, -561.0459) -> (1589.3944, -547.3592)
  line L87 (1593.7078, -543.0459) -> (1623.2875, -543.0459)
  line L88 (1623.2875, -543.0459) -> (1623.2875, -169.0459)
  line L89 (1589.3944, -164.7325) -> (1589.3944, -151.0459)
  line L90 (1589.3944, -151.0459) -> (1539.3944, -151.0459)
  line L91 (1539.3944, -151.0459) -> (1539.3944, -164.7325)
  line L92 (1397.2949, -133.0458) -> (1367.7152, -133.0458)
  line L93 (1367.7152, -133.0458) -> (1367.7152, -507.0458)
  line L94 (1367.7152, -507.0458) -> (1397.2949, -507.0458)
  line L95 (1401.6083, -511.3592) -> (1401.6083, -525.0458)
  line L96 (1401.6083, -525.0458) -> (1451.6083, -525.0458)
  line L97 (1451.6083, -525.0458) -> (1451.6083, -511.3592)
  line L98 (1455.9216, -507.0458) -> (1485.5013, -507.0458)
  line L99 (1485.5013, -507.0458) -> (1485.5013, -133.0458)
  line L100 (1451.6083, -128.7325) -> (1451.6083, -115.0458)
  line L101 (1451.6083, -115.0458) -> (1401.6083, -115.0458)
  line L102 (1401.6083, -115.0458) -> (1401.6083, -128.7325)
  line L103 (1053.7684, -547.2721) -> (1332.7152, -386.2221)
  arc A6 (1332.7152, -386.2221) -> (1332.7152, -334.2606) centre (1317.7152, -360.2413) ccw
  line L104 (1332.7152, -334.2606) -> (1053.7684, -173.2105)
  arc A7 (1053.7684, -173.2105) -> (1008.7684, -199.1913) centre (1038.7684, -199.1913) ccw
  line L105 (1008.7684, -199.1913) -> (1008.7684, -521.2913)
  arc A8 (1008.7684, -521.2913) -> (1053.7684, -547.2721) centre (1038.7684, -521.2913) ccw
  line L106 (1147.0999, -396.4003) -> (1155.3907, -391.6136)
  line L107 (1161.2828, -393.1924) -> (1182.0695, -429.196)
  line L108 (1180.4907, -435.0881) -> (1172.1999, -439.8748)
  line L109 (1166.3078, -438.296) -> (1145.5211, -402.2924)
  line L110 (1092.7615, -355.4547) -> (1092.7615, -365.028)
  line L111 (1088.4481, -369.3413) -> (1046.8748, -369.3413)
  line L112 (1042.5615, -365.028) -> (1042.5615, -355.4547)
  line L113 (1046.8748, -351.1413) -> (1088.4481, -351.1413)
  line L114 (1155.3907, -328.869) -> (1147.0999, -324.0823)
  line L115 (1145.5211, -318.1902) -> (1166.3078, -282.1867)
  line L116 (1172.1999, -280.6079) -> (1180.4907, -285.3945)
  line L117 (1182.0695, -291.2867) -> (1161.2828, -327.2902)
  line L118 (988.7684, -174.7999) -> (908.6976, -174.7999)
  line L119 (730, -174.7999) -> (730, -584.7999)
  line L120 (730, -584.7999) -> (810.0709, -584.7999)
  line L121 (814.3842, -589.1133) -> (814.3842, -602.7999)
  line L122 (814.3842, -602.7999) -> (904.3842, -602.7999)
  line L123 (904.3842, -602.7999) -> (904.3842, -589.1133)
  line L124 (908.6976, -584.7999) -> (988.7684, -584.7999)
  line L125 (988.7684, -584.7999) -> (988.7684, -174.7999)
  line L126 (904.3842, -170.4866) -> (904.3842, -156.7999)
  line L127 (904.3842, -156.7999) -> (814.3842, -156.7999)
  line L128 (814.3842, -156.7999) -> (814.3842, -170.4866)
  line L129 (908.6976, -118.7999) -> (988.7684, -118.7999)
  line L130 (814.3842, -123.1133) -> (814.3842, -136.7999)
  line L131 (814.3842, -136.7999) -> (904.3842, -136.7999)
  line L132 (904.3842, -136.7999) -> (904.3842, -123.1133)
  line L133 (988.7684, -118.7999) -> (988.7684, 291.2001)
  line L134 (988.7684, 291.2001) -> (908.6976, 291.2001)
  line L135 (904.3842, 295.5134) -> (904.3842, 309.2001)
  line L136 (904.3842, 309.2001) -> (814.3842, 309.2001)
  line L137 (814.3842, 309.2001) -> (814.3842, 295.5134)
  line L138 (810.0709, 291.2001) -> (730, 291.2001)
  line L139 (730, 291.2001) -> (730, -118.7999)
  line L140 (1302.7152, 80.2154) -> (1023.7684, -80.8346)
  arc A9 (1023.7684, -80.8346) -> (1023.7684, -132.7961) centre (1038.7684, -106.8153) ccw
  line L141 (1023.7684, -132.7961) -> (1302.7152, -293.8461)
  arc A10 (1302.7152, -293.8461) -> (1347.7152, -267.8654) centre (1317.7152, -267.8654) ccw
  line L142 (1347.7152, -267.8654) -> (1347.7152, 54.2347)
  arc A11 (1347.7152, 54.2347) -> (1302.7152, 80.2154) centre (1317.7152, 54.2347) ccw
  line L143 (1209.3837, -70.6564) -> (1201.093, -75.443)
  line L144 (1195.2008, -73.8642) -> (1174.4142, -37.8607)
  line L145 (1175.993, -31.9685) -> (1184.2837, -27.1819)
  line L146 (1190.1758, -28.7607) -> (1210.9625, -64.7642)
  line L147 (1263.7221, -111.602) -> (1263.7221, -102.0287)
  line L148 (1268.0355, -97.7153) -> (1309.6088, -97.7153)
  line L149 (1313.9221, -102.0287) -> (1313.9221, -111.602)
  line L150 (1309.6088, -115.9153) -> (1268.0355, -115.9153)
  line L151 (1201.093, -138.1877) -> (1209.3837, -142.9743)
  line L152 (1210.9625, -148.8665) -> (1190.1758, -184.87)
  line L153 (1184.2837, -186.4488) -> (1175.993, -181.6621)
  line L154 (1174.4142, -175.77) -> (1195.2008, -139.7665)
  line L155 (1397.295, 296.9541) -> (1367.7153, 296.9541)
  line L156 (1367.7153, 296.9541) -> (1367.7153, -77.0459)
  line L157 (1367.7153, -77.0459) -> (1397.295, -77.0459)
  line L158 (1401.6084, -81.3592) -> (1401.6084, -95.0459)
  line L159 (1401.6084, -95.0459) -> (1451.6084, -95.0459)
  line L160 (1451.6084, -95.0459) -> (1451.6084, -81.3592)
  line L161 (1455.9217, -77.0459) -> (1485.5014, -77.0459)
  line L162 (1485.5014, -77.0459) -> (1485.5014, 296.9541)
  line L163 (1451.6084, 301.2675) -> (1451.6084, 314.9541)
  line L164 (1451.6084, 314.9541) -> (1401.6084, 314.9541)
  line L165 (1401.6084, 314.9541) -> (1401.6084, 301.2675)
  line L166 (1535.0811, 260.9541) -> (1505.5014, 260.9541)
  line L167 (1505.5014, 260.9541) -> (1505.5014, -113.0459)
  line L168 (1505.5014, -113.0459) -> (1535.0811, -113.0459)
  line L169 (1539.3944, -117.3592) -> (1539.3944, -131.0459)
  line L170 (1539.3944, -131.0459) -> (1589.3944, -131.0459)
  line L171 (1589.3944, -131.0459) -> (1589.3944, -117.3592)
  line L172 (1593.7078, -113.0459) -> (1623.2875, -113.0459)
  line L173 (1623.2875, -113.0459) -> (1623.2875, 260.9541)
  line L174 (1589.3944, 265.2675) -> (1589.3944, 278.9541)
  line L175 (1589.3944, 278.9541) -> (1539.3944, 278.9541)
  line L176 (1539.3944, 278.9541) -> (1539.3944, 265.2675)
  line L177 (1535.0812, 690.9541) -> (1505.5015, 690.9541)
  line L178 (1505.5015, 690.9541) -> (1505.5015, 316.9541)
  line L179 (1505.5015, 316.9541) -> (1535.0812, 316.9541)
  line L180 (1539.3945, 312.6408) -> (1539.3945, 298.9541)
  line L181 (1539.3945, 298.9541) -> (1589.3945, 298.9541)
  line L182 (1589.3945, 298.9541) -> (1589.3945, 312.6408)
  line L183 (1593.7079, 316.9541) -> (1623.2876, 316.9541)
  line L184 (1623.2876, 316.9541) -> (1623.2876, 690.9541)
  line L185 (1589.3945, 695.2675) -> (1589.3945, 708.9541)
  line L186 (1589.3945, 708.9541) -> (1539.3945, 708.9541)
  line L187 (1539.3945, 708.9541) -> (1539.3945, 695.2675)
  line L188 (1397.295, 726.9541) -> (1367.7153, 726.9541)
  line L189 (1367.7153, 726.9541) -> (1367.7153, 352.9541)
  line L190 (1367.7153, 352.9541) -> (1397.295, 352.9541)
  line L191 (1401.6084, 348.6408) -> (1401.6084, 334.9541)
  line L192 (1401.6084, 334.9541) -> (1451.6084, 334.9541)
  line L193 (1451.6084, 334.9541) -> (1451.6084, 348.6408)
  line L194 (1455.9217, 352.9541) -> (1485.5014, 352.9541)
  line L195 (1485.5014, 352.9541) -> (1485.5014, 726.9541)
  line L196 (1451.6084, 731.2675) -> (1451.6084, 744.9541)
  line L197 (1451.6084, 744.9541) -> (1401.6084, 744.9541)
  line L198 (1401.6084, 744.9541) -> (1401.6084, 731.2675)
  line L199 (1172.2, 226.2442) -> (1180.4907, 221.4575)
  line L200 (1182.0695, 215.5654) -> (1161.2829, 179.5619)
  line L201 (1155.3907, 177.9831) -> (1147.1, 182.7697)
  line L202 (1145.5212, 188.6619) -> (1166.3078, 224.6654)
  line L203 (1180.4907, 71.7639) -> (1172.2, 66.9773)
  line L204 (1166.3078, 68.5561) -> (1145.5212, 104.5596)
  line L205 (1147.1, 110.4518) -> (1155.3907, 115.2384)
  line L206 (1161.2829, 113.6596) -> (1182.0695, 77.6561)
  line L207 (1042.5615, 141.8241) -> (1042.5615, 151.3974)
  line L208 (1046.8749, 155.7107) -> (1088.4482, 155.7107)
  line L209 (1092.7615, 151.3974) -> (1092.7615, 141.8241)
  line L210 (1088.4482, 137.5107) -> (1046.8749, 137.5107)
  arc A12 (1332.7153, 120.63) -> (1332.7153, 172.5915) centre (1317.7153, 146.6107) ccw
  line L211 (1332.7153, 172.5915) -> (1053.7685, 333.6415)
  arc A13 (1053.7685, 333.6415) -> (1008.7685, 307.6608) centre (1038.7685, 307.6608) ccw
  line L212 (1008.7685, 307.6608) -> (1008.7685, -14.4393)
  arc A14 (1008.7685, -14.4393) -> (1053.7685, -40.42) centre (1038.7685, -14.4393) ccw
  line L213 (1053.7685, -40.42) -> (1332.7153, 120.63)
  line L214 (1184.2838, 320.4032) -> (1175.9931, 325.1899)
  line L215 (1174.4143, 331.082) -> (1195.2009, 367.0856)
  line L216 (1201.0931, 368.6644) -> (1209.3838, 363.8777)
  line L217 (1210.9626, 357.9856) -> (1190.176, 321.982)
  line L218 (1175.9931, 474.8835) -> (1184.2838, 479.6701)
  line L219 (1190.176, 478.0913) -> (1210.9626, 442.0878)
  line L220 (1209.3838, 436.1957) -> (1201.0931, 431.409)
  line L221 (1195.2009, 432.9878) -> (1174.4143, 468.9913)
  line L222 (1313.9223, 404.8233) -> (1313.9223, 395.25)
  line L223 (1309.6089, 390.9367) -> (1268.0356, 390.9367)
  line L224 (1263.7223, 395.25) -> (1263.7223, 404.8233)
  line L225 (1268.0356, 409.1367) -> (1309.6089, 409.1367)
  arc A15 (1023.7685, 426.0174) -> (1023.7685, 374.0559) centre (1038.7685, 400.0367) ccw
  line L226 (1023.7685, 374.0559) -> (1302.7153, 213.0059)
  arc A16 (1302.7153, 213.0059) -> (1347.7153, 238.9867) centre (1317.7153, 238.9867) ccw
  line L227 (1347.7153, 238.9867) -> (1347.7153, 561.0867)
  arc A17 (1347.7153, 561.0867) -> (1302.7153, 587.0675) centre (1317.7153, 561.0867) ccw
  line L228 (1302.7153, 587.0675) -> (1023.7685, 426.0174)
  line L229 (1053.7685, 466.4325) -> (1332.7154, 627.4826)
  arc A18 (1332.7154, 627.4826) -> (1332.7154, 679.4441) centre (1317.7154, 653.4633) ccw
  line L230 (1332.7154, 679.4441) -> (1053.7685, 840.4941)
  arc A19 (1053.7685, 840.4941) -> (1008.7685, 814.5133) centre (1038.7685, 814.5133) ccw
  line L231 (1008.7685, 814.5133) -> (1008.7685, 492.4133)
  arc A20 (1008.7685, 492.4133) -> (1053.7685, 466.4325) centre (1038.7685, 492.4133) ccw
  line L232 (1147.1001, 617.3043) -> (1155.3908, 622.091)
  line L233 (1161.2829, 620.5122) -> (1182.0696, 584.5087)
  line L234 (1180.4908, 578.6165) -> (1172.2001, 573.8299)
  line L235 (1166.3079, 575.4087) -> (1145.5213, 611.4122)
  line L236 (1092.7616, 658.25) -> (1092.7616, 648.6767)
  line L237 (1088.4482, 644.3633) -> (1046.875, 644.3633)
  line L238 (1042.5616, 648.6767) -> (1042.5616, 658.25)
  line L239 (1046.875, 662.5633) -> (1088.4482, 662.5633)
  line L240 (1155.3908, 684.8356) -> (1147.1001, 689.6223)
  line L241 (1145.5213, 695.5144) -> (1166.3079, 731.518)
  line L242 (1172.2001, 733.0968) -> (1180.4908, 728.3101)
  line L243 (1182.0696, 722.418) -> (1161.2829, 686.4144)
  line L244 (908.6976, 347.2001) -> (988.7684, 347.2001)
  line L245 (988.7684, 347.2001) -> (988.7684, 757.2001)
  line L246 (988.7684, 757.2001) -> (908.6976, 757.2001)
  line L247 (904.3842, 761.5134) -> (904.3842, 775.2001)
  line L248 (904.3842, 775.2001) -> (814.3842, 775.2001)
  line L249 (814.3842, 775.2001) -> (814.3842, 761.5134)
  line L250 (810.0709, 757.2001) -> (730, 757.2001)
  line L251 (730, 757.2001) -> (730, 347.2001)
  line L252 (814.3842, 342.8867) -> (814.3842, 329.2001)
  line L253 (814.3842, 329.2001) -> (904.3842, 329.2001)
  line L254 (904.3842, 329.2001) -> (904.3842, 342.8867)
  line L255 (700, -1519.2) -> (1920, -1519.2)
  line L256 (1920, -1519.2) -> (1920, 919.2)
  line L257 (1920, 919.2) -> (700, 919.2)
  line L258 (700, 919.2) -> (700, -1519.2)
  arc A21 (818.5975, -1035.5793) -> (814.2842, -1039.8927) centre (816.4409, -1037.736) ccw
  arc A22 (904.4842, -1039.8927) -> (900.1708, -1035.5793) centre (902.3275, -1037.736) ccw
  arc A23 (900.1708, -1053.7793) -> (904.4842, -1049.466) centre (902.3275, -1051.6226) ccw
  arc A24 (814.2842, -1049.466) -> (818.5975, -1053.7793) centre (816.4409, -1051.6226) ccw
  arc A25 (1048.7422, -1121.357) -> (1042.8501, -1119.7783) centre (1045.7961, -1120.5676) ccw
  arc A26 (1087.9501, -1197.8937) -> (1089.5289, -1192.0016) centre (1088.7395, -1194.9477) ccw
  arc A27 (1073.7672, -1201.1016) -> (1079.6593, -1202.6804) centre (1076.7133, -1201.891) ccw
  arc A28 (1034.5593, -1124.5649) -> (1032.9805, -1130.457) centre (1033.7699, -1127.511) ccw
  arc A29 (1079.6593, -886.6783) -> (1073.7672, -888.257) centre (1076.7133, -887.4676) ccw
  arc A30 (1089.5289, -897.357) -> (1087.9501, -891.4649) centre (1088.7395, -894.411) ccw
  arc A31 (1042.8501, -969.5804) -> (1048.7422, -968.0016) centre (1045.7961, -968.791) ccw
  arc A32 (1032.9805, -958.9016) -> (1034.5593, -964.7937) centre (1033.7699, -961.8477) ccw
  arc A33 (1350.3546, -1210.8132) -> (1344.4624, -1209.2344) centre (1347.4085, -1210.0238) ccw
  arc A34 (1369.5624, -1252.7088) -> (1371.1412, -1246.8167) centre (1370.3518, -1249.7628) ccw
  arc A35 (1355.3796, -1255.9167) -> (1361.2717, -1257.4955) centre (1358.3257, -1256.7061) ccw
  arc A36 (1336.1717, -1214.021) -> (1334.5929, -1219.9132) centre (1335.3823, -1216.9671) ccw
  arc A37 (1334.5929, -1357.8225) -> (1336.1717, -1363.7146) centre (1335.3823, -1360.7685) ccw
  arc A38 (1361.2717, -1320.2401) -> (1355.3796, -1321.8189) centre (1358.3257, -1321.0295) ccw
  arc A39 (1371.1412, -1330.9189) -> (1369.5624, -1325.0268) centre (1370.3518, -1327.9729) ccw
  arc A40 (1344.4624, -1368.5013) -> (1350.3546, -1366.9225) centre (1347.4085, -1367.7119) ccw
  arc A41 (1428.2143, -1279.7678) -> (1423.9009, -1284.0812) centre (1426.0576, -1281.9245) ccw
  arc A42 (1474.1009, -1284.0812) -> (1469.7876, -1279.7678) centre (1471.9442, -1281.9245) ccw
  arc A43 (1469.7876, -1297.9678) -> (1474.1009, -1293.6545) centre (1471.9442, -1295.8111) ccw
  arc A44 (1423.9009, -1293.6545) -> (1428.2143, -1297.9678) centre (1426.0576, -1295.8111) ccw
  arc A45 (1611.7871, -1092.8866) -> (1616.1005, -1097.2) centre (1613.9438, -1095.0433) ccw
  arc A46 (1557.4738, -1097.2) -> (1561.7871, -1092.8866) centre (1559.6304, -1095.0433) ccw
  arc A47 (1561.7871, -1475.5133) -> (1557.4738, -1471.2) centre (1559.6304, -1473.3566) ccw
  arc A48 (1616.1005, -1471.2) -> (1611.7871, -1475.5133) centre (1613.9438, -1473.3566) ccw
  line L259 (1616.1005, -1471.2) -> (1645.6802, -1471.2)
  arc A49 (1611.7872, -662.8866) -> (1616.1006, -667.2) centre (1613.9439, -665.0433) ccw
  arc A50 (1557.4739, -667.2) -> (1561.7872, -662.8866) centre (1559.6305, -665.0433) ccw
  arc A51 (1561.7872, -1045.5133) -> (1557.4739, -1041.2) centre (1559.6305, -1043.3566) ccw
  arc A52 (1616.1006, -1041.2) -> (1611.7872, -1045.5133) centre (1613.9439, -1043.3566) ccw
  line L260 (1645.6803, -667.2) -> (1616.1006, -667.2)
  arc A53 (1419.6879, -563.046) -> (1424.0012, -558.7326) centre (1421.8445, -560.8893) ccw
  arc A54 (1424.0012, -941.3593) -> (1419.6879, -937.046) centre (1421.8445, -939.2026) ccw
  arc A55 (1478.3146, -937.046) -> (1474.0012, -941.3593) centre (1476.1579, -939.2026) ccw